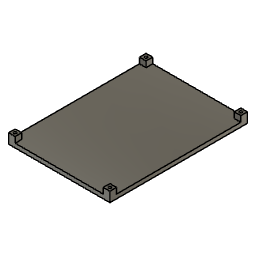
Screen Cover v13 (Autodesk Fusion 360 design; units mm, degrees)
Autodesk Fusion 360 part; units mm, degrees
sketch "Sketch1" plane through (0, 0, 0) normal (0, 0, 1) x (1, 0, 0)
  line L0 (0, 0) -> (122.7, 0)
  line L1 (122.7, 0) -> (122.7, 166.5)
  line L2 (122.7, 166.5) -> (0, 166.5)
  line L3 (0, 166.5) -> (0, 0)
  dimension "d1" = 166.5
  dimension "d2" = 122.7
  constraint horizontal L0
  constraint vertical L1
  constraint horizontal L2
  constraint vertical L3
  constraint coincident L0.start L3.end
  measures "d1" distance of L0.start L2.end
  measures "d2" distance of L0.start L0.end
extrude "Extrude1" add sketch "Sketch1" along normal blind 5
sketch "Sketch2" plane through (0, 0, 5) normal (0, 0, 1) x (-1, 0, 0)
  line L0 (0, -166.5) -> (0, 0)
  line L1 (0, 0) -> (-122.7, 0)
  line L2 (-122.7, 0) -> (-122.7, -166.5)
  line L3 (-122.7, -166.5) -> (0, -166.5)
  line L4 (0, -166.5) -> (-8, -166.5)
  line L5 (-8, -166.5) -> (-8, -158.5)
  line L6 (-8, -158.5) -> (0, -158.5)
  line L7 (0, -158.5) -> (0, -166.5)
  line L8 (0, 0) -> (-8, 0)
  line L9 (-8, 0) -> (-8, -8)
  line L10 (-8, -8) -> (0, -8)
  line L11 (0, -8) -> (0, 0)
  dimension "d5" = 8
  dimension "d6" = 8
  dimension "d7" = 8
  dimension "d8" = 8
  constraint horizontal L4
  constraint vertical L5
  constraint horizontal L6
  constraint vertical L7
  constraint coincident L0.start L3.end
  constraint horizontal L8
  constraint vertical L9
  constraint horizontal L10
  constraint vertical L11
  constraint coincident L0.end L1.start
  measures "d5" distance of L8.end L9.end
  measures "d6" distance of L9.end L10.end
  measures "d7" distance of L5.end L6.end
  measures "d8" distance of L4.end L5.end
extrude "Extrude2" add sketch "Sketch2" along normal blind 7 contours L0 L3 L4 L5 L6 L7 | L0 L1 L8 L9 L10 L11
ref_plane "WorkPlane1" through (61.35, 83.25, 6) normal (-1, 0, 0) x (0, -1, 0)
mirror "Mirror1" about plane through (61.35, 83.25, 6) normal (-1, 0, 0) of "Extrude2"
sketch "Sketch3" plane through (0, 0, 12) normal (0, 0, 1) x (-1, 0, 0)
  line L0 (0, -158.5) -> (-8, -158.5)
  line L1 (-8, -158.5) -> (-8, -166.5)
  line L2 (-8, -166.5) -> (0, -166.5)
  line L3 (0, -166.5) -> (0, -158.5)
  circle A0 centre (-4, -162.5) radius 1.6
  circle A1 centre (-4, -4) radius 1.6
  line L4 (-8, -8) -> (0, -8)
  line L5 (0, -8) -> (0, 0)
  dimension "d13" = 3.2
  dimension "d14" = 4
  dimension "d15" = 4
  dimension "d16" = 3.2
  dimension "d17" = 4
  dimension "d18" = 4
  measures "d13" diameter of A0
  measures "d14" distance of L2 A0.centre
  measures "d15" distance of L1 A0.centre
  measures "d16" diameter of A1
  measures "d17" distance of A1.centre L4
  measures "d18" distance of A1.centre L5
extrude "Extrude3" cut sketch "Sketch3" against normal blind 13 contours A0 | A1
mirror "Mirror2" about plane through (61.35, 83.25, 6) normal (-1, 0, 0) of "Extrude3"
sketch "Sketch4" plane through (0, 0, 0) normal (0, 0, -1) x (1, 0, 0)
  circle A0 centre (118.7, -4) radius 1.6
  circle A1 centre (118.7, -162.5) radius 1.6
  circle A2 centre (4, -4) radius 1.6
  circle A3 centre (4, -162.5) radius 1.6
  line L0 (0, 0) -> (0, -166.5)
  line L1 (0, -166.5) -> (122.7, -166.5)
  line L2 (122.7, -166.5) -> (122.7, 0)
  line L3 (122.7, 0) -> (0, 0)
  circle A4 centre (63.7, -28.5) radius 2.15
  circle A5 centre (112.7, -28.5) radius 2.15
  circle A6 centre (63.7, -86.5) radius 2.15
  circle A7 centre (112.7, -86.5) radius 2.15
  line L4 (60.7, -31.5) -> (66.7, -31.5)
  line L5 (66.7, -31.5) -> (66.7, -25.5)
  line L6 (66.7, -25.5) -> (60.7, -25.5)
  line L7 (60.7, -25.5) -> (60.7, -31.5)
  line L8 (109.7, -25.5) -> (115.7, -25.5)
  line L9 (115.7, -25.5) -> (115.7, -31.5)
  line L10 (115.7, -31.5) -> (109.7, -31.5)
  line L11 (109.7, -31.5) -> (109.7, -25.5)
  line L12 (60.7, -83.5) -> (66.7, -83.5)
  line L13 (66.7, -83.5) -> (66.7, -89.5)
  line L14 (66.7, -89.5) -> (60.7, -89.5)
  line L15 (60.7, -89.5) -> (60.7, -83.5)
  line L16 (109.7, -83.5) -> (115.7, -83.5)
  line L17 (115.7, -83.5) -> (115.7, -89.5)
  line L18 (115.7, -89.5) -> (109.7, -89.5)
  line L19 (109.7, -89.5) -> (109.7, -83.5)
  dimension "d23" = 4.3
  dimension "d24" = 4.3
  dimension "d25" = 4.3
  dimension "d26" = 4.3
  dimension "d27" = 49
  dimension "d28" = 58
  dimension "d29" = 10
  dimension "d30" = 80
  dimension "d39" = 6
  dimension "d40" = 6
  dimension "d41" = 3
  dimension "d42" = 3
  dimension "d43" = 3
  dimension "d44" = 3
  dimension "d45" = 6
  dimension "d46" = 6
  dimension "d47" = 6
  dimension "d48" = 6
  dimension "d49" = 3
  dimension "d51" = 6
  dimension "d52" = 6
  dimension "d53" = 3
  constraint horizontal A4.centre A5.centre
  constraint vertical A5.centre A7.centre
  constraint vertical A4.centre A6.centre
  constraint horizontal A6.centre A7.centre
  constraint horizontal L4
  constraint vertical L5
  constraint horizontal L6
  constraint vertical L7
  constraint horizontal L8
  constraint vertical L9
  constraint horizontal L10
  constraint vertical L11
  constraint horizontal L12
  constraint vertical L13
  constraint horizontal L14
  constraint vertical L15
  constraint horizontal L16
  constraint vertical L17
  constraint horizontal L18
  constraint vertical L19
  measures "d23" diameter of A4
  measures "d24" diameter of A5
  measures "d25" diameter of A6
  measures "d26" diameter of A7
  measures "d27" distance of A4.centre A5.centre
  measures "d28" distance of A5.centre A7.centre
  measures "d29" distance of L2 A5.centre
  measures "d30" distance of L1 A7.centre
  measures "d39" distance of L5.end L6.end
  measures "d40" distance of L4.end L5.end
  measures "d41" distance of A4.centre L6
  measures "d42" distance of A4.centre L7
  measures "d43" distance of A5.centre L8
  measures "d44" distance of A5.centre L11
  measures "d45" distance of L9.end L10.end
  measures "d46" distance of L8.end L9.end
  measures "d47" distance of L12.start L12.end
  measures "d48" distance of L12.end L13.end
  measures "d49" distance of A6.centre L15
  measures "d51" distance of L16.start L16.end
  measures "d52" distance of L16.start L18.end
  measures "d53" distance of A7.centre L19
extrude "Extrude4" cut sketch "Sketch4" against normal blind 3.3 contours A4 | A5 | A6 | A7
sketch "Sketch5" plane through (0, 0, 0) normal (0, 0, -1) x (1, 0, 0)
  circle A0 centre (118.7, -4) radius 1.6
  circle A1 centre (118.7, -162.5) radius 1.6
  circle A2 centre (4, -4) radius 1.6
  circle A3 centre (4, -162.5) radius 1.6
  line L0 (0, 0) -> (0, -166.5)
  line L1 (0, -166.5) -> (122.7, -166.5)
  line L2 (122.7, -166.5) -> (122.7, 0)
  line L3 (122.7, 0) -> (0, 0)
  circle A4 centre (4, -4) radius 2.5
  circle A5 centre (118.7, -4) radius 2.5
  circle A6 centre (118.7, -162.5) radius 2.5
  circle A7 centre (4, -162.5) radius 2.5
  circle A8 centre (63.7, -86.5) radius 2.15
  circle A9 centre (112.7, -28.5) radius 2.15
  circle A10 centre (112.7, -86.5) radius 2.15
  circle A11 centre (63.7, -28.5) radius 2.15
  dimension "d33" = 5
  dimension "d34" = 5
  dimension "d35" = 5
  dimension "d36" = 5
  constraint concentric A2 A4
  constraint concentric A0 A5
  constraint concentric A1 A6
  constraint concentric A3 A7
  measures "d33" diameter of A7
  measures "d34" diameter of A6
  measures "d35" diameter of A5
  measures "d36" diameter of A4
extrude "Extrude5" cut sketch "Sketch5" against normal blind 10 contours A4 | A5 | A6 | A7
equation "d1 = 168.3 mm - 1.8 mm"
equation "d2 = 124 mm - 1.3 mm"
